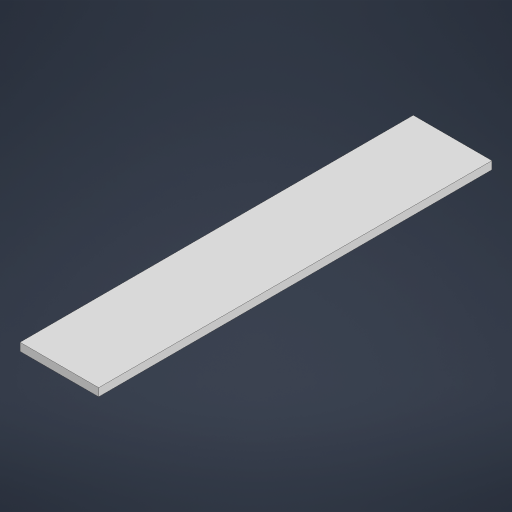
# Autodesk Inventor part: part1
Saved by Autodesk Inventor 2024 (Build 280153000, 153)
## iProperties
Created: 2024-01-20
Part Number: part1
Material: Generic
Document SubType Name: Modeling
Designer: marco
Density: 1 g/cm^3
Appearance: Default
Author: marco
Autodesk Inventor part; units mm, degrees
ref_plane "YZ Plane" through (0, 0, 0) normal (1, 0, 0) x (0, 1, 0)
ref_plane "XZ Plane" through (0, 0, 0) normal (0, 1, 0) x (-1, 0, 0)
ref_plane "XY Plane" through (0, 0, 0) normal (0, 0, 1) x (1, 0, 0)
sketch "Sketch1" plane through (0, 0, 0) normal (0, 1, 0) x (-1, 0, 0)
  line L0 (10.9508, 51.9341) -> (-9.0492, 51.9341)
  line L1 (-9.0492, 51.9341) -> (-9.0492, -48.0659)
  line L2 (-9.0492, -48.0659) -> (10.9508, -48.0659)
  line L3 (10.9508, -48.0659) -> (10.9508, 51.9341)
  line L4 (26.5167, 1.9341) -> (-24.615, 1.9341)
  line L5 (0.9508, 45.2898) -> (0.9508, -41.4217)
  point P0 (0.9508, 1.9341)
  dimension "d1" = 20
  dimension "d2" = 100
  constraints: 12 end point, 3 horizontal, 2 midpoint, 2 parallel, 2 vertical, 1 perpendicular, 2 other
  measures "d1" distance between parallel lines of L1 L3
  measures "d2" distance between parallel lines of L2 L0
extrude "Extrusion1" add sketch "Sketch1" along normal blind 2
body "Solid1"
